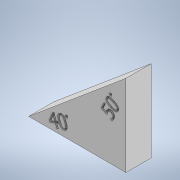
# Autodesk Inventor part: 40-50-DegreeAngleTemplate
Saved by Autodesk Inventor 2020.2 (Build 242310000, 310)
## iProperties
Created: 2020-01-27
Part Number: 40-50-DegreeAngleTemplate
Material: Generic
Document SubType Name: Modeling
Designer: robst
Density: 1 g/cm^3
Appearance: Default
Author: robst
Autodesk Inventor part; units mm, degrees
ref_plane "YZ Plane" through (0, 0, 0) normal (1, 0, 0) x (0, 1, 0)
ref_plane "XZ Plane" through (0, 0, 0) normal (0, 1, 0) x (-1, 0, 0)
ref_plane "XY Plane" through (0, 0, 0) normal (0, 0, 1) x (1, 0, 0)
sketch "Sketch1" plane through (0, 0, 0) normal (0, 0, 1) x (1, 0, 0)
  line L0 (0, 0) -> (97.2876, 81.634)
  line L1 (0, 0) -> (127, 0) construction
  line L2 (97.2876, 81.634) -> (97.2876, 0)
  line L3 (97.2876, 0) -> (0, 0)
  dimension "d0" = 127
  dimension "d1" = 40
  constraints: 8 end point, 1 equal length, 1 horizontal, 1 perpendicular, 1 vertical
  measures "d0" distance of L0.start L0.end
  measures "d1" angle of L1 L0
extrude "Extrusion1" add sketch "Sketch1" along normal mid plane 25.4
sketch "Sketch2" plane through (0, 0, 12.7) normal (0, 0, 1) x (1, 0, 0)
  line L0 (0, 0) -> (97.2876, 0) construction
  line L1 (0, 0) -> (97.2876, 35.4098) construction
  line L2 (97.2876, 0) -> (97.2876, 81.634) construction
  line L3 (29.7312, 8.7075) -> (28.3096, 8.1901)
  line L4 (28.3096, 8.1901) -> (29.8021, 4.0895)
  line L5 (29.8021, 4.0895) -> (28.2644, 3.5299)
  line L6 (28.2644, 3.5299) -> (26.7719, 7.6304)
  line L7 (26.7719, 7.6304) -> (21.5012, 5.712)
  line L8 (21.5012, 5.712) -> (20.8887, 7.3948)
  line L9 (20.8887, 7.3948) -> (23.9884, 15.4886)
  line L10 (23.9884, 15.4886) -> (25.4584, 16.0236)
  line L11 (25.4584, 16.0236) -> (27.8414, 9.4763)
  line L12 (27.8414, 9.4763) -> (29.2631, 9.9938)
  line L13 (29.2631, 9.9938) -> (29.7312, 8.7075)
  line L14 (26.3037, 8.9166) -> (24.6071, 13.5781)
  line L15 (24.6071, 13.5781) -> (22.2902, 7.4559)
  line L16 (22.2902, 7.4559) -> (26.3037, 8.9166)
  spline S0 degree 2 poles (37.7558, 13.742) (38.9245, 10.5312) (38.1527, 6.8442) (36.2088, 6.1366) knots 0 0 0 1 2 2 2
  spline S1 degree 2 poles (36.2088, 6.1366) (34.2359, 5.4186) (31.2729, 7.812) (30.1289, 10.9551) knots 0 0 0 1 2 2 2
  spline S2 degree 2 poles (30.1289, 10.9551) (28.9532, 14.1852) (29.7321, 17.8529) (31.6856, 18.564) knots 0 0 0 1 2 2 2
  spline S3 degree 2 poles (31.6856, 18.564) (33.6488, 19.2785) (36.6224, 16.8561) (37.7558, 13.742) knots 0 0 0 1 2 2 2
  spline S4 degree 2 poles (37.0291, 9.3594) (37.0465, 10.0339) (36.5781, 11.9224) (36.1311, 13.1506) knots 0 0 0 1 2 2 2
  spline S5 degree 2 poles (36.1311, 13.1506) (35.6841, 14.3789) (34.8324, 16.117) (34.3689, 16.6382) knots 0 0 0 1 2 2 2
  spline S6 degree 2 poles (34.3689, 16.6382) (33.9053, 17.1595) (32.8352, 17.4819) (32.1679, 17.239) knots 0 0 0 1 2 2 2
  spline S7 degree 2 poles (32.1679, 17.239) (31.5005, 16.9961) (30.8686, 16.0542) (30.846, 15.3341) knots 0 0 0 1 2 2 2
  spline S8 degree 2 poles (30.846, 15.3341) (30.826, 14.6368) (31.3277, 12.7166) (31.7536, 11.5464) knots 0 0 0 1 2 2 2
  spline S9 degree 2 poles (31.7536, 11.5464) (32.2112, 10.2892) (32.9784, 8.6627) (33.4692, 8.0966) knots 0 0 0 1 2 2 2
  spline S10 degree 2 poles (33.4692, 8.0966) (33.9266, 7.5622) (35.0302, 7.2081) (35.7266, 7.4616) knots 0 0 0 1 2 2 2
  spline S11 degree 2 poles (35.7266, 7.4616) (36.3842, 7.7009) (37.0161, 8.6428) (37.0291, 9.3594) knots 0 0 0 1 2 2 2
  spline S12 degree 2 poles (38.4763, 17.6439) (37.9694, 17.4594) (36.9953, 17.9137) (36.815, 18.409) knots 0 0 0 1 2 2 2
  spline S13 degree 2 poles (36.815, 18.409) (36.6305, 18.9159) (37.0848, 19.89) (37.5916, 20.0745) knots 0 0 0 1 2 2 2
  spline S14 degree 2 poles (37.5916, 20.0745) (38.087, 20.2548) (39.0611, 19.8005) (39.2456, 19.2937) knots 0 0 0 1 2 2 2
  spline S15 degree 2 poles (39.2456, 19.2937) (39.4259, 18.7983) (38.9716, 17.8242) (38.4763, 17.6439) knots 0 0 0 1 2 2 2
  spline S16 degree 2 poles (37.9564, 19.0723) (37.7375, 18.9926) (37.8172, 18.7738) knots 0 0 0 1 1 1
  spline S17 degree 2 poles (37.8172, 18.7738) (37.8926, 18.5664) (38.1115, 18.6461) knots 0 0 0 1 1 1
  spline S18 degree 2 poles (38.1115, 18.6461) (38.3189, 18.7216) (38.2434, 18.9289) knots 0 0 0 1 1 1
  spline S19 degree 2 poles (38.2434, 18.9289) (38.1637, 19.1478) (37.9564, 19.0723) knots 0 0 0 1 1 1
  dimension "d4" = 20
  constraints: 2 end point, 1 point on line, 1 other
  measures "d4" angle of L1 L0
sketch "Sketch3" plane through (0, 0, 12.7) normal (0, 0, 1) x (1, 0, 0)
  line L0 (97.2876, 81.634) -> (0, 0) construction
  line L1 (97.2876, 81.634) -> (59.2211, 0) construction
  line L2 (0, 0) -> (97.2876, 0) construction
  line L3 (97.2876, 0) -> (97.2876, 81.634) construction
  spline S0 degree 2 poles (83.4064, 46.3863) (84.2365, 45.9992) (85.4064, 44.8064) (85.7026, 44.0778) knots 0 0 0 1 2 2 2
  spline S1 degree 2 poles (85.7026, 44.0778) (85.9987, 43.3492) (85.9308, 41.6207) (85.5133, 40.7253) knots 0 0 0 1 2 2 2
  spline S2 degree 2 poles (85.5133, 40.7253) (85.1305, 39.9045) (84.0187, 38.4698) (83.4555, 38.017) knots 0 0 0 1 2 2 2
  line L4 (83.4555, 38.017) -> (81.8232, 38.7781)
  line L5 (81.8232, 38.7781) -> (81.8754, 38.8901)
  spline S3 degree 2 poles (81.8754, 38.8901) (82.0886, 39.0064) (82.7332, 39.5121) (83.0695, 39.8436) knots 0 0 0 1 2 2 2
  spline S4 degree 2 poles (83.0695, 39.8436) (83.4412, 40.2267) (83.9707, 40.8996) (84.1925, 41.3753) knots 0 0 0 1 2 2 2
  spline S5 degree 2 poles (84.1925, 41.3753) (84.41, 41.8416) (84.483, 42.875) (84.2672, 43.3618) knots 0 0 0 1 2 2 2
  spline S6 degree 2 poles (84.2672, 43.3618) (84.0569, 43.8118) (83.282, 44.5366) (82.6663, 44.8236) knots 0 0 0 1 2 2 2
  spline S7 degree 2 poles (82.6663, 44.8236) (82.0507, 45.1107) (81.1106, 45.1403) (80.7016, 44.9449) knots 0 0 0 1 2 2 2
  spline S8 degree 2 poles (80.7016, 44.9449) (80.2602, 44.7533) (79.5654, 43.8963) (79.2913, 43.3087) knots 0 0 0 1 2 2 2
  spline S9 degree 2 poles (79.2913, 43.3087) (78.9956, 42.6744) (78.6043, 41.3239) (78.5099, 40.9023) knots 0 0 0 1 2 2 2
  line L6 (78.5099, 40.9023) -> (72.5776, 43.6686)
  line L7 (72.5776, 43.6686) -> (75.5222, 49.9833)
  line L8 (75.5222, 49.9833) -> (76.8747, 49.3526)
  line L9 (76.8747, 49.3526) -> (74.6217, 44.521)
  line L10 (74.6217, 44.521) -> (77.6904, 43.09)
  spline S10 degree 2 poles (77.6904, 43.09) (77.7836, 43.3872) (78.0079, 43.9412) (78.1123, 44.1651) knots 0 0 0 1 2 2 2
  spline S11 degree 2 poles (78.1123, 44.1651) (78.5255, 45.0512) (79.3844, 46.1383) (80.0744, 46.4979) knots 0 0 0 1 2 2 2
  spline S12 degree 2 poles (80.0744, 46.4979) (80.7688, 46.8668) (82.3617, 46.8734) (83.4064, 46.3863) knots 0 0 0 1 2 2 2
  spline S13 degree 2 poles (85.4223, 56.1887) (88.519, 54.7447) (90.5804, 51.5918) (89.7062, 49.717) knots 0 0 0 1 2 2 2
  spline S14 degree 2 poles (89.7062, 49.717) (88.8189, 47.8142) (85.0313, 47.4114) (81.9999, 48.825) knots 0 0 0 1 2 2 2
  spline S15 degree 2 poles (81.9999, 48.825) (78.8845, 50.2777) (76.8418, 53.4219) (77.7204, 55.3061) knots 0 0 0 1 2 2 2
  spline S16 degree 2 poles (77.7204, 55.3061) (78.6033, 57.1995) (82.4189, 57.5893) (85.4223, 56.1887) knots 0 0 0 1 2 2 2
  spline S17 degree 2 poles (88.0074, 52.5759) (87.5428, 53.0651) (85.8762, 54.0693) (84.6916, 54.6217) knots 0 0 0 1 2 2 2
  spline S18 degree 2 poles (84.6916, 54.6217) (83.507, 55.1741) (81.6758, 55.8009) (80.9794, 55.8417) knots 0 0 0 1 2 2 2
  spline S19 degree 2 poles (80.9794, 55.8417) (80.283, 55.8826) (79.2984, 55.3538) (78.9982, 54.7102) knots 0 0 0 1 2 2 2
  spline S20 degree 2 poles (78.9982, 54.7102) (78.6981, 54.0666) (78.9173, 52.9537) (79.4105, 52.4285) knots 0 0 0 1 2 2 2
  spline S21 degree 2 poles (79.4105, 52.4285) (79.8894, 51.9213) (81.602, 50.9183) (82.7306, 50.392) knots 0 0 0 1 2 2 2
  spline S22 degree 2 poles (82.7306, 50.392) (83.9432, 49.8266) (85.6358, 49.219) (86.3831, 49.1658) knots 0 0 0 1 2 2 2
  spline S23 degree 2 poles (86.3831, 49.1658) (87.0845, 49.1113) (88.1152, 49.6413) (88.4283, 50.3129) knots 0 0 0 1 2 2 2
  spline S24 degree 2 poles (88.4283, 50.3129) (88.7241, 50.9471) (88.5049, 52.06) (88.0074, 52.5759) knots 0 0 0 1 2 2 2
  spline S25 degree 2 poles (83.1727, 59.4572) (82.9447, 58.9684) (81.9347, 58.6007) (81.457, 58.8235) knots 0 0 0 1 2 2 2
  spline S26 degree 2 poles (81.457, 58.8235) (80.9681, 59.0515) (80.6005, 60.0615) (80.8284, 60.5503) knots 0 0 0 1 2 2 2
  spline S27 degree 2 poles (80.8284, 60.5503) (81.0512, 61.0281) (82.0612, 61.3957) (82.5501, 61.1678) knots 0 0 0 1 2 2 2
  spline S28 degree 2 poles (82.5501, 61.1678) (83.0278, 60.945) (83.3955, 59.9349) (83.1727, 59.4572) knots 0 0 0 1 2 2 2
  spline S29 degree 2 poles (81.795, 60.0996) (81.6966, 59.8885) (81.9077, 59.7901) knots 0 0 0 1 1 1
  spline S30 degree 2 poles (81.9077, 59.7901) (82.1077, 59.6968) (82.2061, 59.9079) knots 0 0 0 1 1 1
  spline S31 degree 2 poles (82.2061, 59.9079) (82.2994, 60.1079) (82.0994, 60.2012) knots 0 0 0 1 1 1
  spline S32 degree 2 poles (82.0994, 60.2012) (81.8883, 60.2996) (81.795, 60.0996) knots 0 0 0 1 1 1
  dimension "d5" = 25
  constraints: 2 end point, 1 point on line, 1 other
  measures "d5" angle of L1 L3
extrude "Extrusion2" cut sketch "Sketch2" against normal blind 2.54
extrude "Extrusion3" cut sketch "Sketch3" against normal blind 2.54
body "Solid1"
